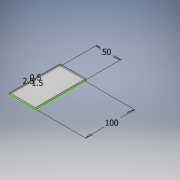
# Autodesk Inventor part: 호출벨 new 커버
Saved by Autodesk Inventor 2019.5 (Build 235369000, 369)
## iProperties
Created: 2021-08-25
Part Number: 호출벨 new 커버
Material: 일반
Document SubType Name: Modeling
Designer: msj19
Density: 1 g/cm^3
Appearance: 기본값
Author: msj19
Autodesk Inventor part; units mm, degrees
ref_plane "우측면도" through (0, 0, 0) normal (1, 0, 0) x (0, 1, 0)
ref_plane "평면도" through (0, 0, 0) normal (0, 1, 0) x (-1, 0, 0)
ref_plane "정면도" through (0, 0, 0) normal (0, 0, 1) x (1, 0, 0)
sketch "스케치1" plane through (0, 0, 0) normal (0, 1, 0) x (-1, 0, 0)
  line L0 (0, 0) -> (0, -100)
  line L1 (0, -100) -> (-50, -100)
  line L2 (-50, -100) -> (-50, 0)
  line L3 (-50, 0) -> (0, 0)
  line L4 (2.5, -102.5) -> (2.5, 2.5)
  line L5 (2.5, 2.5) -> (-52.5, 2.5)
  line L6 (-52.5, 2.5) -> (-52.5, -102.5)
  line L7 (-52.5, -102.5) -> (2.5, -102.5)
  line L8 (1, -101) -> (1, 1)
  line L9 (1, 1) -> (-51, 1)
  line L10 (-51, 1) -> (-51, -101)
  line L11 (-51, -101) -> (1, -101)
  line L12 (1.5, -101.5) -> (1.5, 1.5)
  line L13 (1.5, 1.5) -> (-51.5, 1.5)
  line L14 (-51.5, 1.5) -> (-51.5, -101.5)
  line L15 (-51.5, -101.5) -> (1.5, -101.5)
  dimension "d0" = 50
  dimension "d1" = 100
  dimension "d2" = 2.5
  dimension "d3" = 1.5
  dimension "d4" = 0.5
  constraints: 32 end point, 12 perpendicular, 1 vertical, 9 other
  measures "d0" distance between parallel lines of L2 L0
  measures "d1" distance between parallel lines of L3 L1
  measures "d2" distance between parallel lines of L0 L4
  measures "d3" distance between parallel lines of L0 L12
  measures "d4" distance between parallel lines of L12 L8
extrude "돌출1" add sketch "스케치1" along normal blind 1 contours L0 L1 L2 L3 | L7 L6 L5 L4 | L11 L10 L9 L8 | L15 L14 L13 L12
sketch "스케치2" plane through (0, 1, 0) normal (0, 1, 0) x (1, 0, 0)
  line L0 (51.5, -1.5) -> (51.5, 101.5) projected
  line L1 (51, -1) -> (51, 101) projected
  line L2 (51.5, 101.5) -> (-1.5, 101.5) projected
  line L3 (51, 101) -> (-1, 101) projected
  line L4 (-1.5, 101.5) -> (-1.5, -1.5) projected
  line L5 (-1, 101) -> (-1, -1) projected
  line L6 (-1, -1) -> (51, -1) projected
  line L7 (-1.5, -1.5) -> (51.5, -1.5) projected
  point P0 (0, 0)
extrude "돌출3" add sketch "스케치2" along normal blind 2.5
